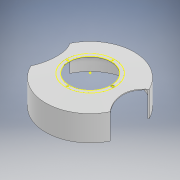
# Autodesk Inventor part: main_protect2
Saved by Autodesk Inventor 2020 (Build 240168000, 168)
## iProperties
Created: 2024-10-23
Part Number: main_protect2
Material: Типовые
Document SubType Name: Modeling
Designer: Ivan
Density: 1 g/cm^3
Appearance: По умолчанию
Author: Ivan
Autodesk Inventor part; units mm, degrees
ref_plane "YZ Plane" through (0, 0, 0) normal (1, 0, 0) x (0, 1, 0)
ref_plane "XZ Plane" through (0, 0, 0) normal (0, 1, 0) x (-1, 0, 0)
ref_plane "XY Plane" through (0, 0, 0) normal (0, 0, 1) x (1, 0, 0)
sketch "Эскиз1" plane through (0, 0, 0) normal (0, 1, 0) x (-1, 0, 0)
  circle A0 centre (0, 0) radius 106.25
  arc A1 (-95.3337, -46.91) -> (-95.3337, 46.91) centre (-154.2365, 0) ccw
  arc A2 (95.3337, 46.91) -> (95.3337, -46.91) centre (154.2365, 0) ccw
  line L0 (-154.2365, 0) -> (154.2365, 0)
  line L1 (-95.3337, 46.91) -> (-55.3337, 46.91) construction
  line L2 (95.3337, 46.91) -> (55.3337, 46.91) construction
  point P0 (74.5593, -32.2924)
  dimension "d5" = 212.5
  dimension "d16" = 75.3
  dimension "d17" = 75.3
  dimension "d18" = 93.82
  dimension "d19" = 40
  dimension "d20" = 93.82
  constraints: 9 point on circle, 6 end point, 3 centre point, 2 coincident, 2 parallel, 1 horizontal, 1 midpoint
  measures "d5" diameter of A0
  measures "d16" radius of A1
  measures "d17" radius of A2
  measures "d18" distance from line of L1 A0.start
  measures "d19" distance of L1.start L1.end
  measures "d20" distance from line of L2 A2.end
sketch "Эскиз2" plane through (0, 0, 0) normal (0, 0, 1) x (1, 0, 0)
  line L0 (106.25, 0) -> (-106.25, 0) projected
  line L1 (106.25, 0) -> (106.25, -70.1)
  line L2 (106.25, -9.1) -> (108.25, -9.1) construction
  line L3 (-149.15, 0) -> (151.15, 0) projected
  line L4 (106.25, -70.1) -> (104.25, -70.1)
  line L5 (104.25, -70.1) -> (104.25, -10.7208)
  line L6 (106.25, -9.1) -> (58.25, 0)
  line L7 (104.25, -10.7208) -> (58.25, -2)
  line L8 (58.25, -2) -> (58.25, 0) construction
  line L9 (50.25, 0) -> (58.25, 0)
  line L10 (50.25, 0) -> (50.25, -2)
  line L11 (50.25, -2) -> (58.25, -2)
  line L12 (0, -84.12) -> (0, 14.02) projected
  point P0 (0, 0)
  dimension "d0" = 70.1
  dimension "d1" = 61
  dimension "d7" = 2
  dimension "d10" = 50.25
  dimension "d11" = 8
  dimension "d34" = 2
  dimension "d35" = 1.965
  constraints: 20 end point, 3 point on line, 3 vertical, 2 perpendicular, 1 horizontal, 1 parallel
  measures "d0" distance of L0.start L1.end
  measures "d1" distance of L2.start L1.end
  measures "d7" distance of L1.end L4.end
  measures "d10" distance of L9.start point (0, 0)
  measures "d11" distance of L6.end L9.start
  measures "d34" distance from line of L9.start L11
  measures "d35" distance from line of L2.start L7
revolve "Вращение1" add sketch "Эскиз2" angle 360 about axis through (0, -10, 0) along (0, 1, 0) contours L6 L1 L4 L5 L7 L11 L10 L0
chamfer "Фаска1" distance 2.5 angle 45 1 edges at (-104.25, -10.7208, 0)
extrude "Выдавливание1" cut sketch "Эскиз1" against normal through all contours L0 A2 A0 | A0 A2 L0 | A1 L0 A0 | A0 L0 A1
sketch "Эскиз3" plane through (0, 0, 0) normal (0, 1, 0) x (1, 0, 0)
  line L0 (148.75, 0) -> (-148.75, 0) construction
  line L1 (0, 148.75) -> (0, -148.75) construction
  circle A0 centre (0, 0) radius 50.25 projected
  circle A1 centre (0, 0) radius 58.25 projected
  circle A2 centre (0, 0) radius 54.25 construction
  circle A3 centre (-54.25, 0) radius 1.65
  circle A4 centre (0, 54.25) radius 1.65
  circle A5 centre (54.25, 0) radius 1.65
  circle A6 centre (0, -54.25) radius 1.65
  point P0 (-50.25, 0)
  point P1 (-58.25, 0)
  dimension "d23" = 8
  dimension "d24" = 4
  dimension "d25" = 3.3
  dimension "d26" = 3.3
  dimension "d27" = 3.3
  dimension "d28" = 3.3
  constraints: 6 point on line, 5 centre point, 4 coincident, 4 point on circle, 2 horizontal alignment, 2 other
  measures "d23" distance of point (-58.25, 0) point (-50.25, 0)
  measures "d24" distance of A2.start point (-50.25, 0)
  measures "d25" diameter of A3
  measures "d26" diameter of A4
  measures "d27" diameter of A5
  measures "d28" diameter of A6
extrude "Выдавливание2" cut sketch "Эскиз3" against normal blind 10 contours A3 | A4 | A5 | A6
sketch "Эскиз4" plane through (0, 0, 0) normal (0, 1, 0) x (1, 0, 0)
  circle A0 centre (54.25, 0) radius 1.65 projected
  circle A1 centre (-54.25, 0) radius 1.65 projected
  circle A2 centre (0, -54.25) radius 1.65 projected
  circle A3 centre (0, 54.25) radius 1.65 projected
  circle A4 centre (0, 0) radius 50.25 projected
  circle A5 centre (0, 0) radius 58.25 projected
chamfer "Фаска2" distance 1.4 angle 45 1 edges at (52.6, 0, 0)
equation "\"d17\" = d16"
equation "\"d20\" = d18"
equation "\"d24\" = 0.5 * d23"
equation "\"d26\" = d25"
equation "\"d27\" = d25"
equation "\"d28\" = d25"
